Cherry holder_v3 (Autodesk Fusion 360 design; units mm, degrees)
Autodesk Fusion 360 part; units mm, degrees
sketch "Sketch1" plane through (0, 0, 0) normal (0, 0, 1) x (1, 0, 0) in component "Component"
  line L0 (150, -15) -> (-150, -15)
  line L1 (-150, -15) -> (-150, 15)
  line L2 (-150, 15) -> (150, 15)
  line L3 (150, 15) -> (150, -15)
  line L4 (150, -15) -> (-150, 15) construction
  line L5 (-150, -15) -> (150, 15) construction
  dimension "d1" = 300
  dimension "d2" = 30
  constraint horizontal L0
  constraint perpendicular L0 L1
  constraint parallel L0 L2
  constraint parallel L1 L3
  constraint coincident L4 origin
  constraint coincident L5 origin
  measures "d1" distance of L1.end L2.end
  measures "d2" distance of L0.end L1.end
extrude "Extrude1" add sketch "Sketch1" along normal blind 30 makes body 1 in component "Component"
sketch "Sketch2" plane through (0, 0, 30) normal (0, 0, 1) x (-1, 0, 0) in component "Component"
  line L0 (-150, -15) -> (150, -15)
  line L1 (150, -15) -> (150, 15)
  line L2 (150, 15) -> (-150, 15)
  line L3 (-150, 15) -> (-150, -15)
  line L4 (-150, 0) -> (-135, 0) construction
  circle A0 centre (-135, 0) radius 6
  circle A1 centre (-105, 0) radius 6
  circle A2 centre (-75, 0) radius 6
  circle A3 centre (-45, 0) radius 6
  circle A4 centre (-15, 0) radius 6
  circle A5 centre (15, 0) radius 6
  circle A6 centre (45, 0) radius 6
  circle A7 centre (75, 0) radius 6
  circle A8 centre (105, 0) radius 6
  circle A9 centre (135, 0) radius 6
  dimension "d5" = 15
  dimension "d6" = 12
  dimension "d9" = 30
  dimension "d10" = 0
  constraint midpoint L3 L4.start
  constraint perpendicular L3 L4
  constraint coincident L4.end A0.centre
  measures "d5" distance of L4.start L4.end
  measures "d6" diameter of A0
extrude "Extrude2" cut sketch "Sketch2" against normal blind 18 contours A0 | A1 | A2 | A3 | A4 | A5 | A6 | A7 | A8 | A9 bodies 1 in component "Component"
chamfer "Chamfer1" distance 10 distance2 10 4 edges at (150, 15, 15) (-150, 15, 15) (-150, -15, 15) (150, -15, 15) measured on face at (150, 5, 10) measured on face at (-50, 15, 10) measured on face at (-150, -5, 10) measured on face at (50, -15, 10) on bodies 1 in component "Component"
sketch "Sketch3" plane through (0, 0, 0) normal (0, 0, -1) x (1, 0, 0) in component "Component"
  line L0 (150, 5) -> (140, 15)
  line L1 (140, 15) -> (-140, 15)
  line L2 (-140, 15) -> (-150, 5)
  line L3 (-150, 5) -> (-150, -5)
  line L4 (-150, -5) -> (-140, -15)
  line L5 (-140, -15) -> (140, -15)
  line L6 (140, -15) -> (150, -5)
  line L7 (150, -5) -> (150, 5)
  line L8 (0, 0) -> (0, 15) construction
  line L9 (0, 15) -> (10, 15) construction
  line L10 (10, 15) -> (-10, -15)
  dimension "d15" = 10
  constraint coincident L8.start origin
  constraint midpoint L1 L8.end
  constraint perpendicular L8 L9
  constraint coincident L5 L10.end
  constraint coincident L8.start L10
  measures "d15" distance of L8.end L9.end
extrude "Extrude3" cut sketch "Sketch3" against normal blind 75 contours L0 L1 L5 L6 L7 L10 bodies 1 in component "Component"
sphere "SpherePrimitive1" add diameter 23 placed x (-1, 0, 0) y (0, -1, 0) z (0, 0, 1) at (-75, 0, 30) separate body makes body 2 in component "Component'"
sketch "Esquisse4" plane through (0, 0, 0) normal (0, 1, 0) x (1, 0, 0) in component "Component"
  line L0 (-9, -30) -> (-21, -30) construction
  line L1 (-15, -30) -> (-15, -51.3107) construction
  circle A0 centre (-15, -39.8107) radius 11.5 construction
  dimension "d21" = 23
  constraint midpoint L0 L1.start
  constraint perpendicular L0 L1
  constraint coincident L0.end A0
  constraint coincident L0.start A0
  constraint coincident L1.end A0
  measures "d21" diameter of A0
component "Component" placed x (1, 0, 0) y (0, 1, 0) z (0, 0, 1) at (0, 0, 0)
component "Component'" placed x (1, 0, 0) y (0, 0, 1) z (0, -1, 0) at (60, 30, 39.8107)
equation "d11 = -( 30 mm - 12 mm )"
